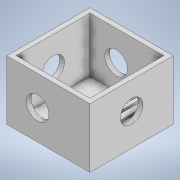
# Autodesk Inventor part: Hülle
Saved by Autodesk Inventor 2021 (Build 250183000, 183)
## iProperties
Created: 2021-01-25
Part Number: Hülle
Material: Generisch
Document SubType Name: Modeling
Designer: Jaro Machnow
Density: 1 g/cm^3
Appearance: Vorgabe
Author: Jaro Machnow
Autodesk Inventor part; units mm, degrees
ref_plane "YZ Plane" through (0, 0, 0) normal (1, 0, 0) x (0, 1, 0)
ref_plane "XZ Plane" through (0, 0, 0) normal (0, 1, 0) x (-1, 0, 0)
ref_plane "XY Plane" through (0, 0, 0) normal (0, 0, 1) x (1, 0, 0)
sketch "Skizze1" plane through (0, 0, 0) normal (0, 1, 0) x (-1, 0, 0)
  line L0 (35, 35) -> (-35, 35)
  line L1 (-35, 35) -> (-35, -35)
  line L2 (-35, -35) -> (35, -35)
  line L3 (35, -35) -> (35, 35)
  line L4 (0, 35) -> (0, -35) construction
  line L5 (35, 0) -> (-35, 0) construction
  point P0 (0, 0)
  point P1 (0, 0)
  dimension "d0" = 70
  dimension "d1" = 70
  constraints: 12 end point, 5 midpoint, 2 parallel, 1 coincident, 1 horizontal, 1 perpendicular
  measures "d0" distance of L2.end L1.end
  measures "d1" distance of L1.end L0.end
extrude "Extrusion1" add sketch "Skizze1" along normal blind 50
shell "Wandung1" thickness 4 removed faces 1 at (11.6667, 50, -11.6667)
sketch "Skizze2" plane through (35, 0, 35) normal (1, 0, 0) x (0, 0, -1)
  circle A0 centre (35, 27) radius 9.5
  line L0 (0, 0) -> (0, 50) construction
  line L1 (0, 0) -> (70, 0) construction
  line L2 (0, 50) -> (70, 0) construction
  line L3 (0, 50) -> (70, 50) construction
  line L4 (70, 50) -> (0, 0) construction
  point P0 (35, 0)
  point P1 (35, 25)
  point P2 (35, 25)
  dimension "d5" = 19
  dimension "d27" = 2
  constraints: 4 end point, 2 midpoint, 1 centre point, 1 vertical alignment
  measures "d5" diameter of A0
  measures "d27" distance of A0.centre point (35, 25)
sketch "Skizze3" plane through (35, 0, -35) normal (0, 0, -1) x (-1, 0, 0)
  circle A0 centre (44, 25) radius 9.5
  line L0 (0, 0) -> (0, 50) construction
  line L1 (70, 0) -> (70, 50) construction
  line L2 (0, 50) -> (70, 0) construction
  line L3 (0, 50) -> (70, 50) construction
  line L4 (0, 0) -> (70, 50) construction
  point P0 (35, 0)
  point P1 (35, 25)
  point P2 (35, 25)
  dimension "d6" = 19
  dimension "d11" = 9
  constraints: 4 end point, 2 midpoint, 1 centre point, 1 horizontal alignment
  measures "d6" diameter of A0
  measures "d11" distance of A0.centre point (35, 25)
extrude "Extrusion2" cut sketch "Skizze3" against normal blind 95.5
extrude "Extrusion3" cut sketch "Skizze2" against normal blind 10
sketch "Skizze4" plane through (-31, 4, -31) normal (0, 1, 0) x (1, 0, 0)
  line L0 (62, -62) -> (0, -62) projected
  line L1 (62, 0) -> (0, 0) projected
  line L2 (62, -62) -> (46, -62)
  line L3 (46, -62) -> (46, 0)
  line L4 (46, 0) -> (62, 0)
  line L5 (62, 0) -> (62, -62)
  point P0 (31, -31)
  dimension "d12" = 16
  constraints: 8 end point, 2 parallel, 1 horizontal, 1 perpendicular, 1 point on line
  measures "d12" distance of L3.end L4.end
extrude "Extrusion4" add sketch "Skizze4" along normal blind 11
sketch "Skizze5" plane through (-31, 15, -31) normal (0, 1, 0) x (1, 0, 0)
  line L0 (62, -62) -> (46, -62) projected
  line L1 (0, 0) -> (62, 0) projected
  line L2 (58, -62) -> (56, -62)
  line L3 (56, -62) -> (56, 0)
  line L4 (56, 0) -> (58, 0)
  line L5 (58, 0) -> (58, -62)
  line L6 (51, -62) -> (49, -62)
  line L7 (49, -62) -> (49, 0)
  line L8 (49, 0) -> (51, 0)
  line L9 (51, 0) -> (51, -62)
  line L10 (62, 0) -> (62, -62) projected
  line L11 (46, 0) -> (46, -62) projected
  line L12 (53.5, -62) -> (53.5, 0) construction
  point P0 (31, -31)
  point P1 (51, 0)
  point P2 (49, 0)
  point P3 (58, 0)
  dimension "d15" = 2
  dimension "d19" = 7.5
  dimension "d20" = 5
  constraints: 18 end point, 6 point on line, 4 parallel, 3 perpendicular, 2 horizontal, 2 other
  measures "d15" distance of L3.end L4.end
  measures "d19" distance between parallel lines of L11 L12
  measures "d20" distance between parallel lines of L3 L9
extrude "Extrusion5" cut sketch "Skizze5" against normal blind 3 contours L0 L3 L1 L5 | L0 L7 L1 L9
fillet "Rundung1" radius 1 4 edges at (27, 12, 0) (25, 12, 0) (20, 12, 0) (18, 12, 0)
sketch "Skizze6" plane through (-35, 0, -35) normal (-1, 0, 0) x (0, 0, 1)
  line L0 (70, 0) -> (70, 50) construction
  line L1 (70, 50) -> (0, 0) construction
  line L2 (0, 0) -> (70, 0) construction
  line L3 (70, 0) -> (0, 50) construction
  circle A0 centre (35, 25) radius 9.5
  point P0 (35, 0)
  dimension "d24" = 19
  constraints: 4 end point, 1 centre point, 1 midpoint
  measures "d24" diameter of A0
extrude "Extrusion6" cut sketch "Skizze6" against normal blind 10
